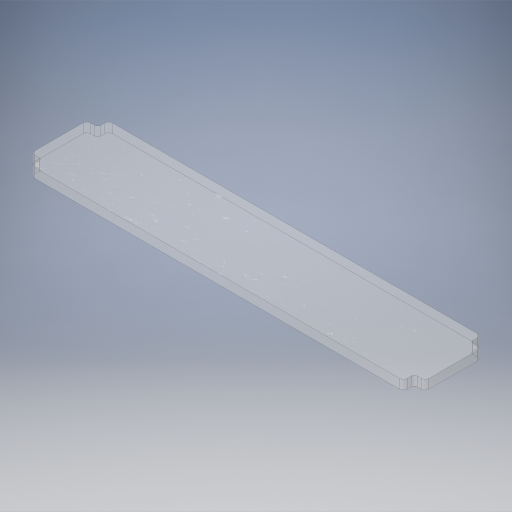
# Autodesk Inventor part: BT704_trajan20_21
Saved by Autodesk Inventor 2023 (Build 270158000, 158)
## iProperties
Company: HTBLA Kaindorf
RuleStatus: InUse
Created: 2022-08-21
Part Number: BT704_trajan20_21
Project: Zeichenmaschine_v2
Material: Acryl
Description: Plexi_220x30
Document SubType Name: Modeling
Designer: trajan20
Density: 1.188 g/cm^3
Appearance: Transparent - farblos
Mass: 51.5952 g
Surface Area: 198.589 cm^2
Volume: 43.4303 cm^3
AfterDocNew0: iProperties-Editor_aufrufen
Author: jan
Keywords: 2021
Autodesk Inventor part; units mm, degrees
ref_plane "YZ Plane" through (0, 0, 0) normal (1, 0, 0) x (0, 1, 0)
ref_plane "XZ Plane" through (0, 0, 0) normal (0, 1, 0) x (-1, 0, 0)
ref_plane "XY Plane" through (0, 0, 0) normal (0, 0, 1) x (1, 0, 0)
derived "BT000_trajan20_22_Zeichenmaschine_neu_Masterskizze.ipt"
sketch "Skizze3" plane through (0, 0, 0) normal (0, 0, 1) x (1, 0, 0)
  line L0 (0, 0) -> (-30, 0)
  line L1 (-30, 0) -> (-30, 200)
  line L2 (-30, 200) -> (0, 200)
  line L3 (0, 200) -> (0, 0)
  line L4 (-30, 200) -> (-35.85, 200)
  line L5 (-35.85, 200) -> (-35.85, 100)
  line L6 (-35.85, 100) -> (-30, 100)
  line L7 (-30, 100) -> (-30, 200)
  line L8 (-30, 200) -> (-15, 200)
  line L9 (-15, 200) -> (-15, 205.85)
  line L10 (-15, 205.85) -> (-30, 205.85)
  line L11 (-30, 205.85) -> (-30, 200)
  dimension "d4" = 200
  dimension "d5" = 30
  dimension "d6" = 5.85
  dimension "d8" = 5.85
  constraints: 24 end point, 6 parallel, 4 point on line, 3 horizontal, 3 perpendicular, 2 midpoint
  measures "d4" distance between parallel lines of L0 L2
  measures "d5" distance between parallel lines of L1 L3
  measures "d6" distance between parallel lines of L2 L10
  measures "d8" distance between parallel lines of L5 L1
extrude "Extrusion3" add sketch "Skizze3" along normal blind 5 contours L0 L1 L2 L3
extrude "Extrusion4" add sketch "Skizze3" along normal blind 5 contours L6 L5 L4 L1 | L2 L11 L10 L9
fillet "Rundung1" radius 2 2 edges at (-35.85, 200, 2.5) (-30, 205.85, 2.5)
mirror "Spiegeln1" about plane through (-15, 200, 0) normal (1, 0, 0) of "Extrusion4", "Rundung1"
mirror "Spiegeln2" about plane through (5.85, 100, 0) normal (0, -1, 0) of "Extrusion4", "Rundung1", "Spiegeln1"
fillet "Rundung2" radius 1.5 4 edges at (0, 0, 2.5) (-30, 0, 2.5) (-30, 200, 2.5) (0, 200, 2.5)
equation "\"d4\" = Basis_Zubau_Länge_Profillänge"
equation "\"d5\" = Basis_Zubau_Höhe_Profillänge - 4 * AluProfil_Abstand"
equation "\"d8\" = d6"
equation "\"Basis_Zubau_Länge_Profillänge\" = 200"
equation "\"Basis_Zubau_Höhe_Profillänge\" = 70"
equation "\"AluProfil_Abstand\" = 10"
